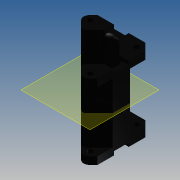
# Autodesk Inventor part: dual stepper mount
Saved by Autodesk Inventor 2013 (Build 170138000, 138)
## iProperties
Created: 2017-03-29
Part Number: dual stepper mount
Material: Generic
Document SubType Name: Modeling
Designer: employee
Density: 1 g/cm^3
Author: employee
Autodesk Inventor part; units mm, degrees
ref_plane "YZ Plane" through (0, 0, 0) normal (1, 0, 0) x (0, 1, 0)
ref_plane "XZ Plane" through (0, 0, 0) normal (0, 1, 0) x (-1, 0, 0)
ref_plane "XY Plane" through (0, 0, 0) normal (0, 0, 1) x (1, 0, 0)
sketch "Sketch1" plane through (0, 0, 0) normal (0, 0, 1) x (1, 0, 0)
  line L0 (-15.5, 15.5) -> (15.5, 15.5) construction
  line L1 (15.5, 15.5) -> (15.5, -15.5) construction
  line L2 (15.5, -15.5) -> (-15.5, -15.5) construction
  line L3 (-15.5, -15.5) -> (-15.5, 15.5) construction
  line L4 (-21, 21) -> (21, 21)
  line L5 (21, 21) -> (21, -21)
  line L6 (21, -21) -> (-21, -21)
  line L7 (-21, -21) -> (-21, 21)
  circle A0 centre (-15.5, 15.5) radius 1.75
  circle A1 centre (15.5, 15.5) radius 1.75
  circle A2 centre (15.5, -15.5) radius 1.75
  circle A3 centre (0, 0) radius 11.25
  dimension "d0" = 31
  dimension "d1" = 42
  dimension "d2" = 22.5
  dimension "d3" = 3.5
  constraints: 16 end point, 6 coincident, 4 centre point, 2 equal radius, 2 horizontal, 18 other
  measures "d0" distance of L0.start L0.end
  measures "d1" distance of L4.start L4.end
  measures "d2" diameter of A3
  measures "d3" diameter of A0
extrude "Extrusion1" add sketch "Sketch1" along normal blind 5
sketch "Sketch2" plane through (0, 0, 5) normal (0, 0, 1) x (1, 0, 0)
  circle A0 centre (15.5, -15.5) radius 1.75 projected
  circle A1 centre (15.5, 15.5) radius 1.75 projected
  circle A2 centre (-15.5, 15.5) radius 1.75 projected
  line L0 (21, 21) -> (-21, 21) projected
  line L1 (-21, 21) -> (-21, -21) projected
  line L2 (-21, -21) -> (21, -21) projected
  line L3 (21, -21) -> (21, 21) projected
  line L4 (-21, 5.7574) -> (-5.7574, 21)
  line L5 (-5.7574, 21) -> (5.7574, 21)
  line L6 (5.7574, 21) -> (21, 5.7574)
  line L7 (21, 5.7574) -> (21, -5.7574)
  line L8 (21, -5.7574) -> (5.7574, -21)
  line L9 (5.7574, -21) -> (2.2218, -17.4645)
  line L10 (2.2218, -17.4645) -> (16, -3.6863)
  line L11 (16, -3.6863) -> (16, 3.6863)
  line L12 (16, 3.6863) -> (3.6863, 16)
  line L13 (3.6863, 16) -> (-3.6863, 16)
  line L14 (-3.6863, 16) -> (-17.4645, 2.2218)
  line L15 (-17.4645, 2.2218) -> (-21, 5.7574)
  dimension "d6" = 5
  dimension "d8" = 3
  dimension "d9" = 5
  dimension "d10" = 3
  dimension "d11" = 45
  dimension "d12" = 5
  dimension "d13" = 5
  dimension "d14" = 3
  constraints: 24 end point, 6 point on line, 4 parallel, 4 perpendicular, 2 collinear
  measures "d6" distance of L8.end L9.end
  measures "d8" distance from line of L8 A0.centre
  measures "d9" distance between parallel lines of L11 L7
  measures "d10" distance from line of L6 A1.centre
  measures "d11" angle of L2 L8
  measures "d12" distance between parallel lines of L6 L12
  measures "d13" distance between parallel lines of L13 L5
  measures "d14" distance from line of L4 A2.centre
extrude "Extrusion2" add sketch "Sketch2" along normal blind 40 contours L6 L3 L8 L9 L10 L11 L12 L13 L14 L15 L4 L0
sketch "Sketch3" plane through (0, 0, 5) normal (0, 0, 1) x (1, 0, 0)
  line L0 (5.7574, -21) -> (2.2218, -17.4645) projected
  line L1 (2.2218, -17.4645) -> (16, -3.6863) projected
  line L2 (16, -3.6863) -> (16, 3.6863) projected
  line L3 (16, 3.6863) -> (3.6863, 16) projected
  line L4 (3.6863, 16) -> (-3.6863, 16) projected
  line L5 (-3.6863, 16) -> (-17.4645, 2.2218) projected
  line L6 (-17.4645, 2.2218) -> (-21, 5.7574) projected
  line L7 (-21, 5.7574) -> (-21, -21) projected
  line L8 (-21, -21) -> (5.7574, -21) projected
  circle A0 centre (0, 0) radius 11.25 projected
extrude "Extrusion3" cut sketch "Sketch3" against normal through all
sketch "Sketch4" plane through (0, 0, 45) normal (0, 0, 1) x (1, 0, 0)
  line L0 (-21, 5.7574) -> (-17.4645, 2.2218) projected
  line L1 (-17.4645, 2.2218) -> (-3.6863, 16) projected
  line L2 (-3.6863, 16) -> (3.6863, 16) projected
  line L3 (3.6863, 16) -> (16, 3.6863) projected
  line L4 (16, 3.6863) -> (16, -3.6863) projected
  line L5 (16, -3.6863) -> (2.2218, -17.4645) projected
  line L6 (2.2218, -17.4645) -> (5.7574, -21) projected
  line L7 (5.7574, -21) -> (21, -5.7574) projected
  line L8 (21, -5.7574) -> (21, 5.7574) projected
  line L9 (21, 5.7574) -> (5.7574, 21) projected
  line L10 (5.7574, 21) -> (-5.7574, 21) projected
  line L11 (-5.7574, 21) -> (-21, 5.7574) projected
  circle A0 centre (-15.5, 15.5) radius 1.75 projected
  line L12 (-21, 5.7574) -> (-5.7574, 21) projected
  line L13 (-5.7574, 21) -> (-21, 21) projected
  line L14 (-21, 21) -> (-21, 5.7574) projected
  circle A1 centre (15.5, 15.5) radius 1.75 projected
  line L15 (5.7574, 21) -> (21, 5.7574) projected
  line L16 (21, 5.7574) -> (21, 21) projected
  line L17 (21, 21) -> (5.7574, 21) projected
  line L18 (21, -5.7574) -> (5.7574, -21) projected
  line L19 (5.7574, -21) -> (21, -21) projected
  line L20 (21, -21) -> (21, -5.7574) projected
  circle A2 centre (15.5, -15.5) radius 1.75 projected
  point P0 (0, 0)
extrude "Extrusion4" add sketch "Sketch4" along normal blind 5
chamfer "Chamfer1" distance 5 angle 45 6 edges at (21, -21, 2.5) (21, -21, 47.5) (21, 21, 47.5) (-21, 21, 47.5) (-21, 21, 2.5) (21, 21, 2.5)
fillet "Fillet3" radius 5.5 4 edges at (16, -3.6863, 25) (16, 3.6863, 25) (3.6863, 16, 25) (-3.6863, 16, 25)
sketch "Sketch5" plane through (0, 0, 50) normal (0, 0, 1) x (1, 0, 0)
  line L0 (21, -16) -> (21, 16) projected
  line L1 (16, 21) -> (-16, 21) projected
  line L2 (21, 5) -> (0, 5)
  line L3 (0, 5) -> (0, -5)
  line L4 (0, -5) -> (21, -5)
  line L5 (21, -5) -> (21, 5)
  line L6 (-5, 21) -> (5, 21)
  line L7 (5, 21) -> (5, 0)
  line L8 (5, 0) -> (-5, 0)
  line L9 (-5, 0) -> (-5, 21)
  point P0 (0, 0)
  point P1 (21, 0)
  point P2 (0, 21)
  point P3 (0, 0)
  dimension "d27" = 10
  constraints: 16 end point, 6 midpoint, 4 parallel, 3 perpendicular, 2 horizontal, 2 point on line, 1 coincident
  measures "d27" distance of L7.end L8.end
extrude "Extrusion5" cut sketch "Sketch5" against normal blind 2.5
ref_plane "Work Plane1" through (0, 0, 25) normal (0, 0, 1) x (1, 0, 0)
mirror "Mirror1" about plane through (0, 0, 25) normal (0, 0, 1) of "Extrusion5"
fillet "Fillet4" radius 2.5 12 edges at (0, 16, 2.5) (-3.3241, 15.6555, 2.5) (3.3241, 15.6555, 2.5) (15.6555, -3.3241, 2.5) (15.6555, 3.3241, 2.5) (16, 0, 2.5) (15.6555, 3.3241, 47.5) (15.6555, -3.3241, 47.5) (16, 0, 47.5) (0, 16, 47.5) (-3.3241, 15.6555, 47.5) (3.3241, 15.6555, 47.5)
sketch "Sketch6" plane through (0, 0, 0) normal (0, 0, -1) x (-1, 0, 0)
  line L0 (5.2972, 14.3891) -> (17.4645, 2.2218) projected
  line L1 (17.4645, 2.2218) -> (21, 5.7574) projected
  line L2 (21, 5.7574) -> (21, 16) projected
  line L3 (-14.6651, -5) -> (-21, -5) projected
  line L4 (-21, -5) -> (-21, -16) projected
  line L5 (-16, -21) -> (-21, -16) projected
  line L6 (-16, -21) -> (-5.7574, -21) projected
  line L7 (-5.7574, -21) -> (-2.2218, -17.4645) projected
  line L8 (-2.2218, -17.4645) -> (-14.3891, -5.2972) projected
  arc A0 (-14.6651, -5) -> (-14.3891, -5.2972) centre (-10.5, -1.4081) ccw projected
  circle A1 centre (-15.5, -15.5) radius 1.75 projected
  line L9 (-14.9995, -21) -> (-6.8429, -12.8434)
  line L10 (12.8434, 6.8429) -> (21, 14.9995)
  point P0 (0, 0)
  constraints: 4 end point, 4 point on line, 2 perpendicular
extrude "Extrusion6" cut sketch "Sketch6" against normal through all contours L10 L2 L1 L0 | L8 L7 L6 L9
fillet "Fillet5" radius 4.24 8 edges at (-21, 14.9995, 2.5) (-21, 16, 2.5) (-21, 14.9995, 47.5) (-21, 16, 47.5) (14.9995, -21, 2.5) (16, -21, 2.5) (16, -21, 47.5) (14.9995, -21, 47.5)
fillet "Fillet6" radius 2.5 4 edges at (-12.8434, 6.8429, 25) (-16.3789, 10.3784, 25) (6.8429, -12.8434, 25) (10.3784, -16.3789, 25)
body "Solid1"
